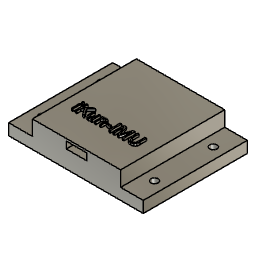
9轴IMU v2 (Autodesk Fusion 360 design; units mm, degrees)
Autodesk Fusion 360 part; units mm, degrees
sketch "草图1" plane through (0, 0, 0) normal (0, 0, 1) x (1, 0, 0)
  line L0 (0, 0) -> (59.5, 0)
  line L1 (59.5, 0) -> (59.5, 46)
  line L2 (59.5, 46) -> (0, 46)
  line L3 (0, 46) -> (0, 0)
  line L4 (-10, 23) -> (68.3933, 23)
  line L5 (29.75, 55) -> (29.75, -17.5748)
  circle A0 centre (5, 36) radius 1.6
  circle A1 centre (54.5, 36) radius 1.6
  circle A2 centre (5, 10) radius 1.6
  circle A3 centre (54.5, 10) radius 1.6
  dimension "d1" = 59.5
  dimension "d2" = 46
  dimension "d3" = 3.2
  dimension "d4" = 49.5
  dimension "d5" = 26
  constraint horizontal L0
  constraint vertical L1
  constraint horizontal L2
  constraint vertical L3
  constraint coincident L0.start L3.end
  constraint perpendicular L1 L4
  constraint vertical L5
  constraint symmetric L1 L3 L5
  constraint symmetric L0 L2 L4
  constraint symmetric L5 A0 A1
  constraint symmetric L4 A0 A2
  constraint symmetric L4 A1 A3
  measures "d1" distance of L0.start L0.end
  measures "d2" distance of L0.start L2.end
  measures "d3" diameter of A0
  measures "d4" distance of A0.centre A1.centre
  measures "d5" distance of A0.centre A2.centre
extrude "拉伸1" add sketch "草图1" along normal blind 5 makes body 1
sketch "草图2" plane through (0, 0, 5) normal (0, 0, 1) x (-1, 0, 0)
  circle A0 centre (-5, -10) radius 1.6
  circle A1 centre (-54.5, -36) radius 1.6
  circle A2 centre (-54.5, -10) radius 1.6
  circle A3 centre (-5, -36) radius 1.6
  line L0 (0, -46) -> (0, 0)
  line L1 (0, 0) -> (-59.5, 0)
  line L2 (-59.5, 0) -> (-59.5, -46)
  line L3 (-59.5, -46) -> (0, -46)
  line L4 (-10.5, -46) -> (-49.5, -46)
  line L5 (-49.5, -46) -> (-49.5, 0)
  line L6 (-49.5, 0) -> (-10.5, 0)
  line L7 (-10.5, 0) -> (-10.5, -46)
  dimension "d8" = 39
  dimension "d9" = 10
  constraint horizontal L4
  constraint vertical L5
  constraint horizontal L6
  constraint vertical L7
  constraint coincident L1 L5.end
  constraint coincident L3 L4.start
  measures "d8" distance of L4.start L4.end
  measures "d9" distance of L2 L5
extrude "拉伸2" add sketch "草图2" along normal blind 6.7 contours L1 L3 L4 L5 L6 L7 bodies 1
sketch "草图3" plane through (0, 0, 0) normal (0, -1, 0) x (1, 0, 0)
  line L0 (0, 0) -> (59.5, 0)
  line L1 (59.5, 0) -> (59.5, 5)
  line L2 (59.5, 5) -> (49.5, 5)
  line L3 (49.5, 5) -> (49.5, 11.7)
  line L4 (49.5, 11.7) -> (10.5, 11.7)
  line L5 (10.5, 11.7) -> (10.5, 5)
  line L6 (10.5, 5) -> (0, 5)
  line L7 (0, 5) -> (0, 0)
  line L8 (25.5, 10.7) -> (34.5, 10.7)
  line L9 (34.5, 10.7) -> (34.5, 7.7)
  line L10 (34.5, 7.7) -> (25.5, 7.7)
  line L11 (25.5, 7.7) -> (25.5, 10.7)
  dimension "d12" = 9
  dimension "d13" = 3
  dimension "d14" = 1
  dimension "d15" = 15
  constraint horizontal L8
  constraint vertical L9
  constraint horizontal L10
  constraint vertical L11
  measures "d12" distance of L8.start L8.end
  measures "d13" distance of L8.start L10.end
  measures "d14" distance of L4 L8
  measures "d15" distance of L3 L9
sketch "草图4" plane through (30, 0, 9.2) normal (0, -1, 0) x (1, 0, 0)
extrude "拉伸3" cut sketch "草图3" against normal blind 9 contours L8 L9 L10 L11 bodies 1
sketch "草图5" plane through (0, 0, 11.7) normal (0, 0, 1) x (-1, 0, 0)
  line L0 (-10.5, 0) -> (-49.5, 0)
  line L1 (-49.5, 0) -> (-49.5, -46)
  line L2 (-49.5, -46) -> (-10.5, -46)
  line L3 (-10.5, -46) -> (-10.5, 0)
  line L4 (-16.0246, -7.6753) -> (-46.2196, -7.6611) construction
  line L5 (-46.2196, -7.6611) -> (-46.2239, -16.8157) construction
  line L6 (-46.2239, -16.8157) -> (-16.0289, -16.8298) construction
  line L7 (-16.0289, -16.8298) -> (-16.0246, -7.6753) construction
  dimension "d18" = 5
  text T0 "iKun-IMU" font "Arial" height 5 align left top in box 30.195 x 9.1545 at (-16.0246, -7.6753) x (-1, 0.000468) y (-0.000468, -1) spacing 1
extrude "拉伸4" add sketch "草图5" along normal blind 1 text T0 bodies 1
copy_body "实体->零部件1" bodies 1 removing the originals makes body 2 in component "Component'"
component "Component'" placed x (1, 0, 0) y (0, 1, 0) z (0, 0, 1) at (0, 0, 0)
